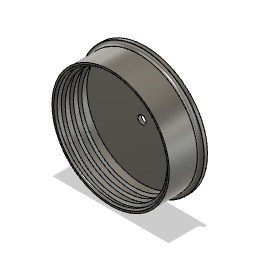
WaterBottleCap_09172021_0842 (Autodesk Fusion 360 design; units mm, degrees)
Autodesk Fusion 360 part; units mm, degrees
sketch "Sketch1" plane through (0, 0, 0) normal (0, 0, 1) x (1, 0, 0)
  circle A0 centre (0, 0) radius 33.375
  dimension "d1" = 66.75
  constraint coincident A0.centre origin
  measures "d1" diameter of A0
extrude "Extrude1" add sketch "Sketch1" along normal blind 15 makes body 1
shell "Shell1" thickness 2 outward yes removed faces 2 at (11.4621, 7.8147, 15) at (11.4621, 7.8147, 0) on bodies 1
coil "CoilPrimitive1" add diameter 66.75 section triangle in size 3 on centre turns 3 pitch 5 right hand placed x (1, 0, 0) y (0, 1, 0) z (0, 0, 1) at (0, 0, 0) separate body makes body 2
extrude "Extrude2" add 1 faces at (34.5766, 1.7575, 15) along direction (0, 0, 1) blind 2 on bodies 1 bodies 1 2
extrude "Extrude3" add 1 faces at (-24.2358, 23.8075, 0) along direction (0, 0, -1) blind 2 on bodies 1 bodies 1
sketch "Sketch4" plane through (0, 0, -2) normal (0, 0, -1) x (-1, 0, 0)
  spline S0 degree 3 poles (19.8575, 28.6696) (16.0566, 31.0858) (11.8237, 32.7421) (3.0267, 34.3141) (-1.4476, 34.2406) (-9.1958, 32.5681) (-12.4708, 31.3064) (-15.4863, 29.5646) knots 0 0 0 0 1.351148 1.351148 2.681785 2.681785 3.730753 3.730753 3.730753 3.730753
  arc A0 (-33.375, 0) -> (-15.4863, 29.5646) centre (0, 0) ccw
  line L0 (-33.375, 0) -> (-34.875, 0)
  arc A1 (19.8575, 28.6696) -> (-34.875, 0) centre (0, 0) ccw
  circle A2 centre (0, 0) radius 35.375
  circle A3 centre (0, 0) radius 37.5
  dimension "d14" = 75
  constraint coincident A0.centre A1.centre
  measures "d14" diameter of A3
extrude "Extrude4" add sketch "Sketch4" along normal blind 2 contours S0 A0 L0 A1 | A2 | A3 bodies 1
sketch "Sketch5" plane through (0, 0, -4) normal (0, 0, -1) x (-1, 0, 0)
  circle A0 centre (0, 0) radius 37.5
  circle A1 centre (0, 0) radius 2.5
  dimension "d17" = 5
  constraint coincident A0.centre A1.centre
  measures "d17" diameter of A1
extrude "Extrude5" cut sketch "Sketch5" against normal blind 11 contours A1 bodies 1
fillet "Fillet3" radius 1 1 edges at (-31.1164, 12.0689, 17) on bodies 1
fillet "Fillet4" radius 2 1 edges at (-32.9811, 12.7921, -2) on bodies 1
